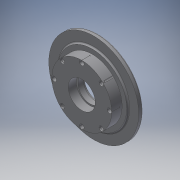
# Autodesk Inventor part: cycloid_outter_motor_side
Saved by Autodesk Inventor 2019.4 (Build 234330000, 330)
## iProperties
Created: 2019-09-11
Part Number: cycloid_outter_motor_side
Material: Generic
Document SubType Name: Modeling
Designer: cdi
Density: 1 g/cm^3
Appearance: Default
Author: cdi
Autodesk Inventor part; units mm, degrees
ref_plane "YZ Plane" through (0, 0, 0) normal (1, 0, 0) x (0, 1, 0)
ref_plane "XZ Plane" through (0, 0, 0) normal (0, 1, 0) x (-1, 0, 0)
ref_plane "XY Plane" through (0, 0, 0) normal (0, 0, 1) x (1, 0, 0)
sketch "Sketch1" plane through (0, 0, 0) normal (0, 0, 1) x (1, 0, 0)
  circle A0 centre (0, 0) radius 14
  circle A1 centre (0, 0) radius 19.96
  dimension "d0" = 28
  dimension "d1" = 39.92
  constraints: 2 centre point, 2 coincident
  measures "d0" diameter of A0
  measures "d1" diameter of A1
extrude "Extrusion1" add sketch "Sketch1" along normal blind 7
sketch "Sketch2" plane through (0, 0, 0) normal (0, 0, -1) x (-1, 0, 0)
  circle A0 centre (0, 0) radius 23
  circle A1 centre (0, 0) radius 14 projected
  dimension "d4" = 46
  constraints: 1 centre point, 1 coincident
  measures "d4" diameter of A0
extrude "Extrusion2" add sketch "Sketch2" along normal blind 6
sketch "Sketch3" plane through (0, 0, 7) normal (0, 0, 1) x (1, 0, 0)
  circle A0 centre (0, 18.42) radius 1.54
  line L0 (0, 0) -> (0, 23.5589)
  circle A1 centre (0, 0) radius 19.96 projected
  dimension "d7" = 3.08
  constraints: 2 end point, 1 centre point, 1 point on line, 1 tangent, 1 vertical
  measures "d7" diameter of A0
extrude "Extrusion3" cut sketch "Sketch3" against normal blind 5.5 contours A0 L0 | L0 A0
pattern_circular "Circular Pattern1" count 8 over 360 about axis through (0, 0, 0) along (0, 0, 1) of "Extrusion3"
sketch "Sketch4" plane through (0, 18.42, 7) normal (0, 0, 1) x (1, 0, 0)
  circle A0 centre (0, -18.42) radius 14 projected
  circle A1 centre (0, -18.42) radius 9.04
  dimension "d14" = 18.08
  constraints: 1 centre point, 1 coincident
  measures "d14" diameter of A1
extrude "Extrusion4" add sketch "Sketch4" against normal blind 11
sketch "Sketch5" plane through (0, 0, -4) normal (0, 0, -1) x (-1, 0, 0)
  circle A0 centre (0, 0) radius 9.04 projected
  circle A1 centre (0, 0) radius 8
  dimension "d17" = 16
  constraints: 1 centre point, 1 coincident
  measures "d17" diameter of A1
extrude "Extrusion5" add sketch "Sketch5" against normal blind 5.5
sketch "Sketch7" plane through (0, 0, -6) normal (0, 0, -1) x (-1, 0, 0)
  circle A0 centre (0, 0) radius 23 projected
  circle A1 centre (0, 0) radius 30
  dimension "d27" = 60
  constraints: 1 centre point, 1 coincident
  measures "d27" diameter of A1
extrude "Extrusion6" add sketch "Sketch7" against normal blind 5
fillet "Fillet1" radius 1 1 edges at (30, 0, -6)
sketch "Sketch8" plane through (0, 0, -6) normal (0, 0, -1) x (-1, 0, 0)
  circle A0 centre (0, 0) radius 22.5
  dimension "d31" = 45
  constraints: 1 centre point, 1 coincident
  measures "d31" diameter of A0
extrude "Extrusion7" cut sketch "Sketch8" against normal blind 2
sketch "Sketch9" plane through (0, 0, -4) normal (0, 0, -1) x (-1, 0, 0)
  circle A0 centre (13.0249, 13.0249) radius 1.54 projected
  circle A1 centre (13.0249, -13.0249) radius 1.54 projected
  circle A2 centre (-13.0249, -13.0249) radius 1.54 projected
  circle A3 centre (-13.0249, 13.0249) radius 1.54 projected
  point P0 (0, 0)
  point P1 (14.1139, 14.1139)
  point P2 (14.1139, -14.1139)
  point P3 (-14.1139, -14.1139)
  point P4 (-14.1139, 14.1139)
  constraints: 4 other
hole "Hole2" at (13.0249, 13.0249, -4) at (-13.0249, 13.0249, -4) at (-13.0249, -13.0249, -4) at (13.0249, -13.0249, -4) direction (0, 0, 1) diameter 3.25 depth 10 countersink diameter 6.5 countersink angle 90
fillet "Fillet3" radius 1 1 edges at (23, 0, -1)
sketch "Sketch10" plane through (0, 0, -6) normal (0, 0, -1) x (-1, 0, 0)
  circle A0 centre (0, 0) radius 39.6905
  constraints: 1 centre point, 1 coincident
extrude "Extrusion8" cut sketch "Sketch10" against normal up to surface (2 mm away)
fillet "Fillet4" radius 1 1 edges at (30, 0, -4)
fillet "Fillet5" radius 2 1 edges at (8, 0, -4)
body "Solid1"
